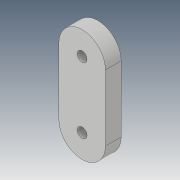
# Autodesk Inventor part: spacer
Saved by Autodesk Inventor 2018 (Build 220112000, 112)
## iProperties
Created: 2020-01-20
Part Number: spacer
Material: Generic
Document SubType Name: Modeling
Designer: anirudh
Density: 1 g/cm^3
Appearance: Default
Author: anirudh
Autodesk Inventor part; units mm, degrees
ref_plane "YZ Plane" through (0, 0, 0) normal (1, 0, 0) x (0, 1, 0)
ref_plane "XZ Plane" through (0, 0, 0) normal (0, 1, 0) x (-1, 0, 0)
ref_plane "XY Plane" through (0, 0, 0) normal (0, 0, 1) x (1, 0, 0)
sketch "Sketch1" plane through (0, 0, 0) normal (0, 0, 1) x (1, 0, 0)
  circle A0 centre (0, 0) radius 1.75
  circle A1 centre (0, 0) radius 8.255
  dimension "d1" = 3.5
  dimension "d4" = 16.51
  constraints: 2 centre point, 1 coincident
  measures "d1" diameter of A0
  measures "d4" diameter of A1
extrude "Extrusion2" add sketch "Sketch1" along normal blind 5.588
sketch "Sketch2" plane through (0, 0, 5.588) normal (0, 0, 1) x (1, 0, 0)
  arc A0 (8.255, 23.4188) -> (-8.255, 23.4188) centre (0, 23.4188) ccw
  line L0 (-8.255, 23.4188) -> (-8.255, 0)
  line L1 (8.255, 23.4188) -> (8.255, 0)
  arc A1 (8.255, 0) -> (-8.255, 0) centre (0, 0) ccw
  circle A2 centre (0, 23.4188) radius 1.75
  dimension "d8" = 16.51
  dimension "d9" = 3.5
  constraints: 4 end point, 4 point on circle, 3 centre point, 2 coincident, 1 parallel, 1 vertical
  measures "d8" diameter of A0
  measures "d9" diameter of A2
extrude "Extrusion3" add sketch "Sketch2" against normal blind 5.588
body "Solid2"
